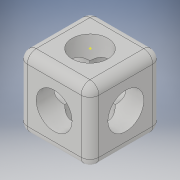
# Autodesk Inventor part: FirstPart
Saved by Autodesk Inventor 2018 (Build 220112000, 112)
## iProperties
Created: 2018-12-12
Part Number: FirstPart
Material: Generic
Document SubType Name: Modeling
Designer: nicholasmantione
Density: 1 g/cm^3
Appearance: Default
Author: nicholasmantione
Autodesk Inventor part; units mm, degrees
ref_plane "YZ Plane" through (0, 0, 0) normal (1, 0, 0) x (0, 1, 0)
ref_plane "XZ Plane" through (0, 0, 0) normal (0, 1, 0) x (-1, 0, 0)
ref_plane "XY Plane" through (0, 0, 0) normal (0, 0, 1) x (1, 0, 0)
sketch "Sketch1" plane through (0, 0, 0) normal (0, 0, 1) x (1, 0, 0)
  line L0 (-12.677, 12.5729) -> (12.723, 12.5729)
  line L1 (12.723, 12.5729) -> (12.723, -12.8271)
  line L2 (12.723, -12.8271) -> (-12.677, -12.8271)
  line L3 (-12.677, -12.8271) -> (-12.677, 12.5729)
  point P0 (0, 0)
  dimension "d0" = 25.4
  dimension "d1" = 25.4
  constraints: 8 end point, 2 parallel, 1 horizontal, 1 perpendicular
  measures "d0" distance of L1.end L2.end
  measures "d1" distance of L0.end L1.end
extrude "Extrusion1" add sketch "Sketch1" along normal blind 25.4
fillet "Fillet1" radius 3.175 12 edges at (0.023, 12.5729, 0) (-12.677, 12.5729, 12.7) (0.023, 12.5729, 25.4) (12.723, 12.5729, 12.7) (12.723, -0.1271, 0) (12.723, -0.1271, 25.4) (12.723, -12.8271, 12.7) (-12.677, -0.1271, 25.4) (0.023, -12.8271, 25.4) (0.023, -12.8271, 0) (-12.677, -0.1271, 0) (-12.677, -12.8271, 12.7)
hole "Hole1" at (0.023, 12.5729, 12.7) direction (0, -1, 0) diameter 12.7 end through all both
hole "Hole2" at (0.023, -0.1271, 0) direction (0, 0, 1) diameter 12.7 end through all
hole "Hole3" at (-12.677, -0.1271, 12.7) direction (1, 0, 0) diameter 12.7 end through all
body "Solid1"
